Autodesk Fusion 360 part; units mm, degrees
(part 2 of 2)
extrude "Extrude14" cut sketch "Sketch13" against normal blind 0.4 text T0 bodies 1
ref_plane "WorkPlane1" through (188.09607, 50.389158, 5.3) normal (-1, 0, 0) x (0, 1, 0)
split "Split1" by plane through (188.09607, 50.389158, 5.3) normal (-1, 0, 0) bodies 1 makes body 2 at (98.189636, 58.471497, -1.4)
sketch "Lock - top down" plane through (0, 0, 0) normal (0, 0, 1) x (-1, 0, 0)
  line L0 (-188.09607, 25.880703) -> (-270.11999, 4.081969)
  line L1 (-188.09607, 25.880703) -> (-188.09607, 24.018221) construction
  line L2 (-145.25227, 37.2669) -> (-188.09607, 25.880703)
  line L3 (-188.09607, -104.43641) -> (-320.63607, -104.43641) construction
  line L4 (-320.63607, -104.43641) -> (-320.63607, -106.23641)
  line L5 (-320.63607, -106.23641) -> (-188.09607, -106.23641)
  line L6 (-188.09607, -104.43641) -> (-188.09607, -106.23641) construction
  line L7 (-115.16607, -106.23641) -> (5.90393, -106.23641)
  line L8 (5.90393, -106.23641) -> (5.90393, -104.43641)
  line L9 (-192.09607, -106.23641) -> (-192.09607, 24.81766)
  line L10 (-184.09607, 26.943745) -> (-184.09607, -106.23641)
  line L11 (-192.09607, -104.23641) -> (-184.09607, -104.23641)
  line L12 (-184.09607, 24.874322) -> (-192.09607, 22.748236)
  line L13 (-270.11999, 4.081969) -> (-269.657669, 2.342355)
  line L14 (-144.789949, 35.527286) -> (-145.25227, 37.2669)
  line L15 (-137.86607, -69.87641) -> (-132.868569, -69.87641)
  line L16 (-124.863571, -69.87641) -> (-119.86607, -69.87641)
  line L17 (-116.96607, -104.43641) -> (-115.16607, -106.23641)
  line L18 (-188.09607, -106.23641) -> (-142.56607, -106.23641)
  line L19 (-142.56607, -106.23641) -> (-140.76607, -104.43641)
  line L20 (-140.76607, -104.43641) -> (-188.09607, -104.43641)
  line L21 (-137.86607, -72.23641) -> (-137.86607, -69.87641)
  line L22 (-119.86607, -72.23641) -> (-137.86607, -72.23641)
  line L23 (-119.86607, -69.87641) -> (-119.86607, -72.23641)
  line L24 (-188.09607, 24.018221) -> (-188.09607, -104.43641)
  line L25 (-188.09607, -104.43641) -> (-140.76607, -104.43641)
  line L26 (-140.76607, -104.43641) -> (-140.56607, -104.23641)
  line L27 (-140.56607, -104.23641) -> (-138.06607, -104.23641)
  line L28 (-138.06607, -104.23641) -> (-138.06607, -106.23641)
  line L29 (-138.06607, -106.23641) -> (-119.66607, -106.23641)
  line L30 (-119.66607, -106.23641) -> (-119.66607, -104.23641)
  line L31 (-119.66607, -104.23641) -> (-117.16607, -104.23641)
  line L32 (-117.16607, -104.23641) -> (-116.96607, -104.43641)
  line L33 (-116.96607, -104.43641) -> (5.90393, -104.43641)
  arc A0 (-112.893785, 35.52631) -> (-113.462504, 35.60109) centre (-113.462504, 33.40109) ccw
  arc A1 (-144.22489, 35.60109) -> (-144.789949, 35.527286) centre (-144.22489, 33.40109) ccw
  line L34 (-144.789949, 35.527286) -> (-188.09607, 24.018221)
  spline S0 degree 3 poles (-112.443833, -34.178821) (-112.623273, -34.494325) (-113.067742, -35.275823) (-113.065754, -36.182515) (-113.064569, -36.72316) knots 0 0 0 0 0.10731568 0.26581945 0.26581945 0.26581945 0.26581945
  line L35 (-113.064569, -36.72316) -> (-113.064569, -42.493965)
  line L36 (-113.064569, -42.493965) -> (-114.387899, -42.493965)
  line L37 (-114.387899, -42.493965) -> (-114.387899, -36.716339)
  spline S1 degree 3 poles (-114.387899, -36.716339) (-114.381596, -36.26218) (-114.370302, -35.448421) (-114.145967, -34.667263) (-114.046834, -34.322069) knots 0 0 0 0 0.13550051 0.24278952 0.24278952 0.24278952 0.24278952
  spline S2 degree 3 poles (-114.046834, -34.322069) (-113.906454, -34.037924) (-113.617939, -33.453933) (-113.087792, -33.074291) (-112.815592, -32.879367) knots 0 0 0 0 0.09355856 0.19228664 0.19228664 0.19228664 0.19228664
  spline S3 degree 3 poles (-112.815592, -32.879367) (-112.478265, -32.717522) (-111.741613, -32.364087) (-110.923037, -32.337723) (-110.479304, -32.323432) knots 0 0 0 0 0.11104148 0.24249104 0.24249104 0.24249104 0.24249104
  spline S4 degree 3 poles (-110.479304, -32.323432) (-110.047361, -32.335898) (-109.250425, -32.358896) (-108.516614, -32.666749) (-108.180531, -32.807744) knots 0 0 0 0 0.12830104 0.23671581 0.23671581 0.23671581 0.23671581
  spline S5 degree 3 poles (-108.180531, -32.807744) (-107.904382, -32.986281) (-107.355446, -33.341181) (-107.054502, -33.921257) (-106.904951, -34.209517) knots 0 0 0 0 0.09682209 0.19246489 0.19246489 0.19246489 0.19246489
  spline S6 degree 3 poles (-106.904951, -34.209517) (-106.793937, -34.568785) (-106.542046, -35.383961) (-106.529805, -36.238445) (-106.52296, -36.716339) knots 0 0 0 0 0.11226089 0.25471982 0.25471982 0.25471982 0.25471982
  line L38 (-106.52296, -36.716339) -> (-106.52296, -42.493965)
  line L39 (-106.52296, -42.493965) -> (-107.846289, -42.493965)
  line L40 (-107.846289, -42.493965) -> (-107.846289, -36.72316)
  spline S7 degree 3 poles (-107.846289, -36.72316) (-107.847634, -36.343348) (-107.84994, -35.692243) (-108.018296, -35.064519) (-108.088444, -34.802969) knots 0 0 0 0 0.11330981 0.19424498 0.19424498 0.19424498 0.19424498
  spline S8 degree 3 poles (-108.088444, -34.802969) (-108.184252, -34.608653) (-108.377047, -34.217634) (-108.738706, -33.973974) (-108.92064, -33.8514) knots 0 0 0 0 0.06380029 0.1283847 0.1283847 0.1283847 0.1283847
  spline S9 degree 3 poles (-108.92064, -33.8514) (-109.135887, -33.754007) (-109.593807, -33.546811) (-110.096788, -33.527429) (-110.363342, -33.517157) knots 0 0 0 0 0.07019817 0.14934107 0.14934107 0.14934107 0.14934107
  spline S10 degree 3 poles (-110.363342, -33.517157) (-110.795816, -33.526901) (-111.560117, -33.544122) (-112.176308, -33.986681) (-112.443833, -34.178821) knots 0 0 0 0 0.12608975 0.22283569 0.22283569 0.22283569 0.22283569
  line L41 (-144.265113, -35.959176) -> (-144.265113, -32.493965)
  line L42 (-144.265113, -32.493965) -> (-142.941785, -32.493965)
  line L43 (-142.941785, -32.493965) -> (-142.941785, -42.493965)
  line L44 (-142.941785, -42.493965) -> (-144.265113, -42.493965)
  line L45 (-144.265113, -42.493965) -> (-144.265113, -37.534892)
  line L46 (-144.265113, -37.534892) -> (-149.23101, -42.493965)
  line L47 (-149.23101, -42.493965) -> (-151.025005, -42.493965)
  line L48 (-151.025005, -42.493965) -> (-146.82992, -38.442123)
  line L49 (-146.82992, -38.442123) -> (-151.209183, -32.493965)
  line L50 (-151.209183, -32.493965) -> (-149.462934, -32.493965)
  line L51 (-149.462934, -32.493965) -> (-145.902224, -37.555356)
  line L52 (-145.902224, -37.555356) -> (-144.265113, -35.959176)
  line L53 (-141.168254, -33.674046) -> (-141.168254, -32.493965)
  line L54 (-141.168254, -32.493965) -> (-133.705771, -32.493965)
  line L55 (-133.705771, -32.493965) -> (-133.705771, -42.493965)
  line L56 (-133.705771, -42.493965) -> (-140.936332, -42.493965)
  line L57 (-140.936332, -42.493965) -> (-140.936332, -41.313883)
  line L58 (-140.936332, -41.313883) -> (-135.029099, -41.313883)
  line L59 (-135.029099, -41.313883) -> (-135.029099, -38.251127)
  line L60 (-135.029099, -38.251127) -> (-140.561161, -38.251127)
  line L61 (-140.561161, -38.251127) -> (-140.561161, -37.077867)
  line L62 (-140.561161, -37.077867) -> (-135.029099, -37.077867)
  line L63 (-135.029099, -37.077867) -> (-135.029099, -33.674046)
  line L64 (-135.029099, -33.674046) -> (-141.168254, -33.674046)
  spline S11 degree 3 poles (-125.397449, -35.386188) (-125.414017, -35.692568) (-125.445705, -36.278547) (-125.747831, -36.780418) (-125.891991, -37.019886) knots 0 0 0 0 0.09046334 0.17301977 0.17301977 0.17301977 0.17301977
  spline S12 degree 3 poles (-125.891991, -37.019886) (-126.079647, -37.223157) (-126.469521, -37.645473) (-127.016751, -37.824189) (-127.300587, -37.916885) knots 0 0 0 0 0.08158021 0.16949141 0.16949141 0.16949141 0.16949141
  spline S13 degree 3 poles (-127.300587, -37.916885) (-127.06715, -38.01369) (-126.628992, -38.195393) (-126.314973, -38.549517) (-126.168254, -38.714974) knots 0 0 0 0 0.07466522 0.14014532 0.14014532 0.14014532 0.14014532
  spline S14 degree 3 poles (-126.168254, -38.714974) (-126.060853, -38.900198) (-125.838394, -39.283854) (-125.813025, -39.727163) (-125.799904, -39.956448) knots 0 0 0 0 0.06330397 0.13112172 0.13112172 0.13112172 0.13112172
  spline S15 degree 3 poles (-125.799904, -39.956448) (-125.832227, -40.30541) (-125.896695, -41.001416) (-126.355554, -41.528538) (-126.584351, -41.791372) knots 0 0 0 0 0.10234001 0.20411691 0.20411691 0.20411691 0.20411691
  spline S16 degree 3 poles (-126.584351, -41.791372) (-126.877698, -42.008074) (-127.496494, -42.46519) (-128.266624, -42.510868) (-128.671665, -42.534892) knots 0 0 0 0 0.1070725 0.22586208 0.22586208 0.22586208 0.22586208
  spline S17 degree 3 poles (-128.671665, -42.534892) (-129.079798, -42.509729) (-129.858761, -42.461704) (-130.482503, -41.996014) (-130.779441, -41.77432) knots 0 0 0 0 0.11969848 0.22845716 0.22845716 0.22845716 0.22845716
  spline S18 degree 3 poles (-130.779441, -41.77432) (-131.012216, -41.507532) (-131.476443, -40.975473) (-131.543898, -40.272717) (-131.57753, -39.922341) knots 0 0 0 0 0.10341204 0.20623613 0.20623613 0.20623613 0.20623613
  spline S19 degree 3 poles (-131.57753, -39.922341) (-131.563978, -39.700323) (-131.537565, -39.267595) (-131.319013, -38.89365) (-131.212592, -38.711564) knots 0 0 0 0 0.06569458 0.12804326 0.12804326 0.12804326 0.12804326
  spline S20 degree 3 poles (-131.212592, -38.711564) (-131.068359, -38.547248) (-130.76111, -38.19722) (-130.331873, -38.014062) (-130.104134, -37.916885) knots 0 0 0 0 0.06475419 0.1379406 0.1379406 0.1379406 0.1379406
  spline S21 degree 3 poles (-130.104134, -37.916885) (-130.388871, -37.806733) (-130.934545, -37.595637) (-131.321072, -37.157687) (-131.505907, -36.948263) knots 0 0 0 0 0.09007569 0.1726221 0.1726221 0.1726221 0.1726221
  spline S22 degree 3 poles (-131.505907, -36.948263) (-131.64613, -36.709971) (-131.93585, -36.217629) (-131.969464, -35.646688) (-131.986809, -35.352081) knots 0 0 0 0 0.08171904 0.16884183 0.16884183 0.16884183 0.16884183
  spline S23 degree 3 poles (-131.986809, -35.352081) (-131.949796, -34.942429) (-131.876151, -34.12734) (-131.344184, -33.505746) (-131.079576, -33.196557) knots 0 0 0 0 0.12016795 0.23909935 0.23909935 0.23909935 0.23909935
  spline S24 degree 3 poles (-131.079576, -33.196557) (-130.743042, -32.942037) (-130.03822, -32.408982) (-129.154103, -32.352792) (-128.692129, -32.323432) knots 0 0 0 0 0.12378696 0.25925417 0.25925417 0.25925417 0.25925417
  spline S25 degree 3 poles (-128.692129, -32.323432) (-128.230062, -32.35299) (-127.345349, -32.409583) (-126.641109, -32.94445) (-126.304679, -33.199967) knots 0 0 0 0 0.13548121 0.25940369 0.25940369 0.25940369 0.25940369
  spline S26 degree 3 poles (-126.304679, -33.199967) (-126.040079, -33.512459) (-125.505218, -34.144126) (-125.433624, -34.969257) (-125.397449, -35.386188) knots 0 0 0 0 0.11970174 0.24196374 0.24196374 0.24196374 0.24196374
  spline S27 degree 3 poles (-118.129372, -32.719068) (-117.841224, -32.865778) (-117.272459, -33.155365) (-116.882486, -33.66027) (-116.690081, -33.909381) knots 0 0 0 0 0.09567893 0.18885751 0.18885751 0.18885751 0.18885751
  spline S28 degree 3 poles (-116.690081, -33.909381) (-116.53669, -34.185253) (-116.225484, -34.744951) (-116.169406, -35.383154) (-116.140968, -35.706788) knots 0 0 0 0 0.09356517 0.18982727 0.18982727 0.18982727 0.18982727
  line L65 (-116.140968, -35.706788) -> (-117.389262, -35.815929)
  spline S29 degree 3 poles (-117.389262, -35.815929) (-117.424475, -35.583463) (-117.490381, -35.148377) (-117.702954, -34.763791) (-117.80195, -34.584688) knots 0 0 0 0 0.06987289 0.13077519 0.13077519 0.13077519 0.13077519
  spline S30 degree 3 poles (-117.80195, -34.584688) (-117.931551, -34.429273) (-118.209, -34.09656) (-118.599824, -33.907701) (-118.808088, -33.807061) knots 0 0 0 0 0.06000975 0.12846872 0.12846872 0.12846872 0.12846872
  spline S31 degree 3 poles (-118.808088, -33.807061) (-119.047244, -33.720546) (-119.542987, -33.54121) (-120.070069, -33.520866) (-120.342877, -33.510336) knots 0 0 0 0 0.07581588 0.15715756 0.15715756 0.15715756 0.15715756
  spline S32 degree 3 poles (-120.342877, -33.510336) (-120.582462, -33.517679) (-121.038692, -33.531663) (-121.473417, -33.669829) (-121.67985, -33.735438) knots 0 0 0 0 0.07150431 0.13616204 0.13616204 0.13616204 0.13616204
  spline S33 degree 3 poles (-121.67985, -33.735438) (-121.857054, -33.812535) (-122.189368, -33.957117) (-122.43029, -34.22686) (-122.542741, -34.352764) knots 0 0 0 0 0.05717377 0.10721873 0.10721873 0.10721873 0.10721873
  spline S34 degree 3 poles (-122.542741, -34.352764) (-122.625305, -34.485598) (-122.78859, -34.748303) (-122.813507, -35.056483) (-122.825825, -35.208835) knots 0 0 0 0 0.04618267 0.09133478 0.09133478 0.09133478 0.09133478
  spline S35 degree 3 poles (-122.825825, -35.208835) (-122.81517, -35.359823) (-122.79418, -35.657239) (-122.632549, -35.907558) (-122.552973, -36.030799) knots 0 0 0 0 0.04460729 0.08786735 0.08786735 0.08786735 0.08786735
  spline S36 degree 3 poles (-122.552973, -36.030799) (-122.437896, -36.14655) (-122.180107, -36.405848) (-121.840545, -36.544231) (-121.652564, -36.62084) knots 0 0 0 0 0.04849047 0.10862537 0.10862537 0.10862537 0.10862537
  spline S37 degree 3 poles (-121.652564, -36.62084) (-121.437712, -36.689718) (-120.851407, -36.877679) (-120.251978, -37.019017) (-119.872209, -37.108561) knots 0 0 0 0 0.0676665 0.18465412 0.18465412 0.18465412 0.18465412
  spline S38 degree 3 poles (-119.872209, -37.108561) (-119.47739, -37.202893) (-118.81705, -37.360665) (-118.192797, -37.626014) (-117.941786, -37.73271) knots 0 0 0 0 0.12148559 0.2031865 0.2031865 0.2031865 0.2031865
  spline S39 degree 3 poles (-117.941786, -37.73271) (-117.721877, -37.85975) (-117.304663, -38.100773) (-117.012447, -38.483037) (-116.874255, -38.663814) knots 0 0 0 0 0.07532125 0.14290023 0.14290023 0.14290023 0.14290023
  spline S40 degree 3 poles (-116.874255, -38.663814) (-116.771798, -38.856053) (-116.564323, -39.245336) (-116.53686, -39.685765) (-116.52296, -39.908698) knots 0 0 0 0 0.06454147 0.1306966 0.1306966 0.1306966 0.1306966
  spline S41 degree 3 poles (-116.52296, -39.908698) (-116.54157, -40.158038) (-116.579167, -40.661749) (-116.827363, -41.10186) (-116.952701, -41.324114) knots 0 0 0 0 0.07402724 0.14954839 0.14954839 0.14954839 0.14954839
  spline S42 degree 3 poles (-116.952701, -41.324114) (-117.116848, -41.532096) (-117.456724, -41.962733) (-117.951828, -42.200498) (-118.207816, -42.323432) knots 0 0 0 0 0.07840025 0.16233219 0.16233219 0.16233219 0.16233219
  spline S43 degree 3 poles (-118.207816, -42.323432) (-118.495607, -42.422882) (-119.089912, -42.628251) (-119.71853, -42.652163) (-120.042741, -42.664496) knots 0 0 0 0 0.09081868 0.18754589 0.18754589 0.18754589 0.18754589
  spline S44 degree 3 poles (-120.042741, -42.664496) (-120.394859, -42.652668) (-121.066727, -42.6301) (-121.701679, -42.410764) (-122.003861, -42.306379) knots 0 0 0 0 0.10500378 0.20035528 0.20035528 0.20035528 0.20035528
  spline S45 degree 3 poles (-122.003861, -42.306379) (-122.268393, -42.176241) (-122.783471, -41.922845) (-123.137789, -41.47186) (-123.310137, -41.25249) knots 0 0 0 0 0.08718517 0.16976088 0.16976088 0.16976088 0.16976088
  spline S46 degree 3 poles (-123.310137, -41.25249) (-123.444931, -41.010775) (-123.718586, -40.520054) (-123.773435, -39.960638) (-123.801267, -39.676774) knots 0 0 0 0 0.082079 0.16663353 0.16663353 0.16663353 0.16663353
  line L66 (-123.801267, -39.676774) -> (-122.532509, -39.581276)
  spline S47 degree 3 poles (-122.532509, -39.581276) (-122.484819, -39.872176) (-122.39501, -40.419999) (-122.017295, -40.824186) (-121.840149, -41.013746) knots 0 0 0 0 0.08618809 0.16231 0.16231 0.16231 0.16231
  spline S48 degree 3 poles (-121.840149, -41.013746) (-121.602465, -41.154557) (-121.067884, -41.47126) (-120.443876, -41.488488) (-120.097312, -41.498057) knots 0 0 0 0 0.081603 0.18353537 0.18353537 0.18353537 0.18353537
  spline S49 degree 3 poles (-120.097312, -41.498057) (-119.742766, -41.492671) (-119.121598, -41.483235) (-118.580085, -41.185766) (-118.347652, -41.058084) knots 0 0 0 0 0.10435003 0.18282243 0.18282243 0.18282243 0.18282243
  spline S50 degree 3 poles (-118.347652, -41.058084) (-118.187557, -40.907924) (-117.878612, -40.61815) (-117.824575, -40.199217) (-117.79854, -39.997375) knots 0 0 0 0 0.06363897 0.12280803 0.12280803 0.12280803 0.12280803
  spline S51 degree 3 poles (-117.79854, -39.997375) (-117.814133, -39.826253) (-117.845034, -39.487143) (-118.073951, -39.235344) (-118.187353, -39.110608) knots 0 0 0 0 0.05006588 0.09921491 0.09921491 0.09921491 0.09921491
  spline S52 degree 3 poles (-118.187353, -39.110608) (-118.413847, -38.984379) (-119.036408, -38.637416) (-119.73692, -38.490959) (-120.182578, -38.397784) knots 0 0 0 0 0.07744908 0.21288227 0.21288227 0.21288227 0.21288227
  spline S53 degree 3 poles (-120.182578, -38.397784) (-120.639459, -38.295711) (-121.390654, -38.127884) (-122.113052, -37.863556) (-122.396083, -37.759994) knots 0 0 0 0 0.14023156 0.2305656 0.2305656 0.2305656 0.2305656
  spline S54 degree 3 poles (-122.396083, -37.759994) (-122.662565, -37.624714) (-123.161966, -37.371191) (-123.518854, -36.940899) (-123.685305, -36.740213) knots 0 0 0 0 0.08854229 0.16593291 0.16593291 0.16593291 0.16593291
  spline S55 degree 3 poles (-123.685305, -36.740213) (-123.806653, -36.523933) (-124.054515, -36.082168) (-124.085559, -35.576221) (-124.101405, -35.317975) knots 0 0 0 0 0.07338817 0.14990011 0.14990011 0.14990011 0.14990011
  spline S56 degree 3 poles (-124.101405, -35.317975) (-124.081323, -35.05419) (-124.04059, -34.519163) (-123.77767, -34.05115) (-123.644378, -33.813883) knots 0 0 0 0 0.07834442 0.15890295 0.15890295 0.15890295 0.15890295
  spline S57 degree 3 poles (-123.644378, -33.813883) (-123.471352, -33.5898) (-123.114605, -33.127785) (-122.597555, -32.85575) (-122.331281, -32.715656) knots 0 0 0 0 0.08389533 0.1729758 0.1729758 0.1729758 0.1729758
  spline S58 degree 3 poles (-122.331281, -32.715656) (-122.031399, -32.601293) (-121.411006, -32.364699) (-120.747206, -32.337489) (-120.40427, -32.323432) knots 0 0 0 0 0.09561639 0.19781016 0.19781016 0.19781016 0.19781016
  spline S59 degree 3 poles (-120.40427, -32.323432) (-119.984393, -32.334089) (-119.205676, -32.353854) (-118.468889, -32.603862) (-118.129372, -32.719068) knots 0 0 0 0 0.12513569 0.23208022 0.23208022 0.23208022 0.23208022
  dimension "d45" = 2
  dimension "d46" = 2
  constraint parallel L5 L11
  constraint parallel L0 L12
  measures "d45" distance of L5 L11
  measures "d46" distance of L0 L12
extrude "Extrude5" add sketch "Lock - top down" along normal blind 1.4 contours L0 L2 L9 L10 L12 L24 L34 | L9 L11 L12 L24 | L10 L12 L24 L34 | L5 L9 L10 L11 L18 L20 L24 L25 | L10 L11 L12 L24 | L10 L11 L20 L24 L25 picked at (-190.762737, 23.792392) picked at (-189.429403, -19.225632) picked at (-185.429403, 24.657936) picked at (-190.762737, -104.969743) picked at (-185.429403, -18.516937) picked at (-186.762737, -104.369743) bodies 1
extrude "Extrude6" add sketch "Lock - top down" along normal up to surface (12 mm away) contours L0 L2 L9 L10 L12 L24 L34 | L10 L12 L24 L34 | L5 L9 L10 L11 L18 L20 L24 L25 | L10 L11 L20 L24 L25 picked at (-190.762737, 23.792392) picked at (-185.429403, 24.657936) picked at (-190.762737, -104.969743) picked at (-186.762737, -104.369743) bodies 1
chamfer "Chamfer2" distance 1.8 angle 45 2 edges at (188.09607, 104.23641, 1.4) (188.09607, -23.811279, 1.4) on bodies 1
combine "Combine1" operation cut target body 1 tool bodies 2 keep tools
sketch "Lock - gap - profile" plane through (184.09607, 0, 0) normal (-1, 0, 0) x (0, -1, 0)
  line L0 (26.943745, 1.8) -> (26.943745, 12)
  line L1 (26.943745, 12) -> (24.874322, 12)
  line L2 (24.874322, 12) -> (24.874322, 3.2)
  line L3 (-106.03641, 12) -> (-106.03641, 1.882843)
  line L4 (-106.03641, 1.882843) -> (-104.353567, 0.2)
  line L5 (-104.353567, 0.2) -> (25.288206, 0.2)
  line L6 (26.643745, 12) -> (26.643745, 1.927273)
  line L7 (26.643745, 1.927273) -> (24.856516, 0.2)
  line L8 (25.081264, 0) -> (26.943745, 1.8)
  line L9 (-104.43641, 0) -> (25.081264, 0)
  line L10 (24.874322, 3.2) -> (23.01184, 1.4)
  line L11 (23.01184, 1.4) -> (-102.43641, 1.4)
  line L12 (-102.43641, 1.4) -> (-104.23641, 3.2)
  line L13 (-104.23641, 3.2) -> (-104.23641, 12)
  line L14 (-104.23641, 12) -> (-106.23641, 12)
  line L15 (-106.23641, 12) -> (-106.23641, 1.8)
  line L16 (-106.23641, 1.8) -> (-104.43641, 0)
  dimension "d63" = 0.3
  constraint parallel L0 L6
  measures "d63" distance of L0 L6
extrude "Extrude8" cut sketch "Lock - gap - profile" against normal up to surface (4 mm away) contours L3 L4 L5 L8 L9 L14 L15 L16 picked at (-18.16621, 0.066667) bodies 1
sweep "Sweep1" cut profiles "Lock - gap - profile" along 1 edges at (186.09607, -26.412224, 12) section 1 contours L0 L1 L5 L6 L7 L8 picked at (26.843745, 5.242424) on bodies 1 bodies 1
equation "d8 = 1.8 mm"
equation "d9 = d8"
equation "d11 = d10"
equation "d12 = d10"
equation "d13 = d10"
equation "d14 = d10"
equation "d15 = d10"
equation "d16 = d10"
equation "d17 = d10"
equation "d21 = d18"
equation "d22 = d18"
equation "d23 = d18"
equation "d24 = d18"
equation "d25 = d18"
equation "d26 = d18"
equation "d27 = d18"
equation "d31 = d30"
equation "d34 = d30"
equation "d35 = d30"
equation "d36 = d30"
equation "d37 = d30"
equation "d38 = d30"
equation "d45 = abs(wall_thickness)"
equation "d46 = abs(wall_thickness)"
equation "d49 = d8"
equation "d74 = 2.65 mm + 2 * 1 mm"
equation "d75 = 8.98 mm + 2 * 0.6 mm"
equation "d98 = 'US8EK'"
named bodies: "Case right", "Case left"
